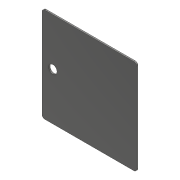
# Autodesk Inventor part: AntennaNameplate
Saved by Autodesk Inventor 2017 (Build 210142000, 142)
## iProperties
Created: 2017-04-20
Part Number: AntennaNameplate
Material: Generic
Document SubType Name: Modeling
Designer: krosie
Density: 1 g/cm^3
Appearance: Anodized - Light Gray
Author: krosie
Autodesk Inventor part; units mm, degrees
ref_plane "YZ Plane" through (0, 0, 0) normal (1, 0, 0) x (0, 1, 0)
ref_plane "XZ Plane" through (0, 0, 0) normal (0, 1, 0) x (-1, 0, 0)
ref_plane "XY Plane" through (0, 0, 0) normal (0, 0, 1) x (1, 0, 0)
sketch "Sketch1" plane through (0, 0, 0) normal (0, 1, 0) x (-1, 0, 0)
  line L0 (-35, 35) -> (35, 35)
  line L1 (35, 35) -> (35, -35)
  line L2 (35, -35) -> (-35, -35)
  line L3 (-35, -35) -> (-35, 35)
  line L4 (-35, 35) -> (35, -35) construction
  line L5 (35, 35) -> (-35, -35) construction
  point P0 (0, 0)
  dimension "d0" = 70
  dimension "d1" = 70
  constraints: 12 end point, 2 midpoint, 2 parallel, 1 horizontal, 1 perpendicular
  measures "d0" distance of L1.end L2.end
  measures "d1" distance of L0.end L1.end
extrude "Extrusion1" add sketch "Sketch1" along normal blind 1
sketch "Sketch2" plane through (0, 1, 0) normal (0, 1, 0) x (1, 0, 0)
  line L0 (-17, -17) -> (-17, 35) construction
  line L1 (25, -35) -> (25, 35) construction
  line L2 (35, -35) -> (35, 35) projected
  line L3 (-35, 35) -> (-35, -35) projected
  line L4 (-10.2536, 14.5438) -> (28, -4.9295)
  line L5 (28, -4.9295) -> (28, -11.3476)
  line L6 (28, -11.3476) -> (-11.7123, 9.2196)
  line L7 (-11.7123, 9.2196) -> (-11.7123, -14.0097)
  line L8 (-11.7123, -14.0097) -> (-17, -14.0097)
  line L9 (-17, -14.0097) -> (-17, 14.5438)
  line L10 (-17, 14.5438) -> (-10.2536, 14.5438)
  point P0 (0, 0)
  dimension "d4" = 10
  dimension "d5" = 18
  constraints: 4 end point, 2 vertical, 1 coincident, 1 point on line, 1 other
  measures "d4" distance between parallel lines of L2 L1
  measures "d5" distance between parallel lines of L3 L0
sketch "Sketch5" plane through (0, 1, 0) normal (0, 1, 0) x (1, 0, 0)
  circle A0 centre (-27, 0) radius 3.1
  line L0 (-35, 35) -> (-35, -35) projected
  line L1 (-35, 0) -> (0, 0) construction
  dimension "d14" = 6.2
  dimension "d15" = 8
  constraints: 2 end point, 1 centre point, 1 horizontal, 1 midpoint, 1 point on line
  measures "d14" diameter of A0
  measures "d15" distance from line of L0 A0.centre
extrude "Extrusion4" cut sketch "Sketch5" against normal up to next
fillet "Fillet1" radius 2 4 edges at (-35, 0.5, -35) (-35, 0.5, 35) (35, 0.5, -35) (35, 0.5, 35)
emboss "Emboss2" sketch "Sketch2" operation cut depth 0.1 direction (0, -1, 0)
body "Solid1"
